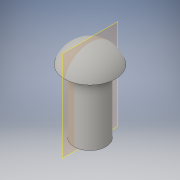
# Autodesk Inventor part: Caufield_Hitch_Peg
Saved by Autodesk Inventor 2016 (Build 200138000, 138)
## iProperties
Created: 2018-01-08
Part Number: Caufield_Hitch_Peg
Material: Generic
Document SubType Name: Modeling
Designer: caufield58738
Density: 1 g/cm^3
Appearance: Default
Mass: 0.585785 g
Surface Area: 4.61173 cm^2
Volume: 0.585785 cm^3
Author: caufield58738
Autodesk Inventor part; units mm, degrees
ref_plane "YZ Plane" through (0, 0, 0) normal (1, 0, 0) x (0, 1, 0)
ref_plane "XZ Plane" through (0, 0, 0) normal (0, 1, 0) x (-1, 0, 0)
ref_plane "XY Plane" through (0, 0, 0) normal (0, 0, 1) x (1, 0, 0)
sketch "Hitch Peg Sketch" plane through (0, 0, 0) normal (0, 0, 1) x (1, 0, 0)
  line L0 (0, 0) -> (0, 16.51)
  line L1 (0, 0) -> (3.175, 0)
  line L2 (3.175, 0) -> (3.175, 12.7)
  line L3 (3.175, 12.7) -> (5.08, 12.7)
  arc A0 (5.08, 12.7) -> (0, 16.51) centre (0.0064, 11.2268) ccw
  dimension "d0" = 16.51
  dimension "d3" = 3.175
  dimension "d4" = 12.7
  dimension "d5" = 1.905
  dimension "d6" = 5.2832
  constraints: 8 end point, 2 point on circle, 2 vertical, 1 centre point, 1 horizontal, 1 perpendicular
  measures "d0" distance of L0.start L0.end
  measures "d3" distance of L0.start L1.end
  measures "d4" distance of L1.end L2.end
  measures "d5" distance of L2.end L3.end
  measures "d6" radius of A0
revolve "Hitch Peg Revolve" add sketch "Hitch Peg Sketch" angle 360 about axis through (0, 0, 0) along (0, 1, 0)
body "Solid1"
